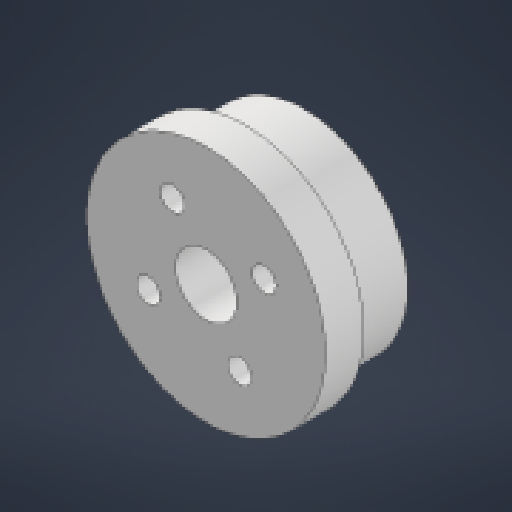
# Autodesk Inventor part: gear_support
Saved by Autodesk Inventor 2026.1 (Build 301233020, 233B)
## iProperties
Created: 2025-11-12
Part Number: gear_support
Material: 일반
Document SubType Name: Modeling
Designer: jaewook
Density: 1 g/cm^3
Appearance: 기본값
Author: jaewook
Autodesk Inventor part; units mm, degrees
ref_plane "YZ Plane" through (0, 0, 0) normal (1, 0, 0) x (0, 1, 0)
ref_plane "XZ Plane" through (0, 0, 0) normal (0, 1, 0) x (-1, 0, 0)
ref_plane "XY Plane" through (0, 0, 0) normal (0, 0, 1) x (1, 0, 0)
sketch "스케치1" plane through (0, 0, 0) normal (0, 0, 1) x (1, 0, 0)
  circle A0 centre (77.7382, 82.3139) radius 1.75 projected
  circle A1 centre (72.7611, 90.8713) radius 1.75 projected
  circle A2 centre (86.2956, 87.2909) radius 1.75 projected
  circle A3 centre (81.3185, 95.8484) radius 1.75 projected
  circle A4 centre (79.5283, 89.0811) radius 11.15 projected
  circle A5 centre (79.5283, 89.0811) radius 10.85
  circle A6 centre (79.5283, 89.0811) radius 1.6
  circle A7 centre (79.5283, 89.0811) radius 2.8
  circle A8 centre (79.5283, 89.0811) radius 2.5 projected
  point P0 (0, 0)
  dimension "d0" = 0.3
  dimension "d3" = 3.2
  constraints: 3 centre point, 1 coincident
  measures "d0" radial gap between concentric circles of A4 A5
  measures "d3" diameter of A6
extrude "돌출1" add sketch "스케치1" along normal blind 13.4 contours A5 | A7 | A8
sketch "스케치2" plane through (79.5283, 89.0811, 13.4) normal (0, 0, 1) x (1, 0, 0)
  circle A0 centre (0, 0) radius 10.85 projected
  circle A1 centre (0, 0) radius 12.5
  dimension "d4" = 25
  constraints: 1 centre point, 1 coincident
  measures "d4" diameter of A1
extrude "돌출2" add sketch "스케치2" against normal blind 4
chamfer "모따기1" distance 0.2 angle 45 1 edges at (68.6783, 89.0811, 0)
sketch "스케치3" plane through (79.5283, 89.0811, 0) normal (0, 0, -1) x (-1, 0, 0)
  circle A0 centre (0, 0) radius 1.6 projected
  circle A1 centre (0, 0) radius 10.65 projected
  circle A2 centre (0, 0) radius 3.2
  dimension "d13" = 6.4
  constraints: 1 centre point, 1 coincident
  measures "d13" diameter of A2
extrude "돌출3" cut sketch "스케치3" against normal blind 12.5 contours A2
sketch "스케치5" plane through (79.5283, 89.0811, 13.4) normal (0, 0, 1) x (1, 0, 0)
  circle A0 centre (0, 0) radius 12.5 projected
  circle A1 centre (-1.7902, -6.7672) radius 1.75 projected
  circle A2 centre (-1.7902, -6.7672) radius 1.25
  circle A3 centre (3.5193, -6.051) radius 1.25
  circle A4 centre (6.7672, -1.7902) radius 1.25
  circle A5 centre (6.051, 3.5193) radius 1.25
  circle A6 centre (1.7902, 6.7672) radius 1.25
  circle A7 centre (-3.5193, 6.051) radius 1.25
  circle A8 centre (-6.7672, 1.7902) radius 1.25
  circle A9 centre (-6.051, -3.5193) radius 1.25
  dimension "d18" = 2.5
  dimension "d21" = 360
  constraints: 8 centre point, 1 coincident, 17 other
  measures "d18" diameter of A2
extrude "돌출5" cut sketch "스케치5" against normal blind 3.5 contours A3 | A5 | A7 | A9
sketch "스케치4" plane through (79.5283, 89.0811, 13.4) normal (0, 0, 1) x (1, 0, 0)
  circle A0 centre (1.7902, 6.7672) radius 1.75 projected
  circle A1 centre (6.7672, -1.7902) radius 1.75 projected
  circle A2 centre (-6.7672, 1.7902) radius 1.75 projected
  circle A3 centre (-1.7902, -6.7672) radius 1.75 projected
extrude "돌출4" add sketch "스케치4" against normal blind 3
